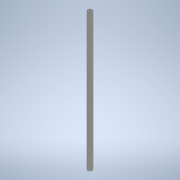
# Autodesk Inventor part: Eje
Saved by Autodesk Inventor 2020.3 (Build 243373000, 373)
## iProperties
Created: 2020-07-24
Part Number: Eje
Material: Stainless Steel
Document SubType Name: Modeling
Designer: juanp
Density: 8 g/cm^3
Appearance: Semi-Polished
Author: juanp
Autodesk Inventor part; units mm, degrees
ref_plane "YZ Plane" through (0, 0, 0) normal (1, 0, 0) x (0, 1, 0)
ref_plane "XZ Plane" through (0, 0, 0) normal (0, 1, 0) x (-1, 0, 0)
ref_plane "XY Plane" through (0, 0, 0) normal (0, 0, 1) x (1, 0, 0)
sketch "Sketch1" plane through (0, 0, 0) normal (0, 1, 0) x (-1, 0, 0)
  circle A0 centre (0, 0) radius 2.5
  dimension "d0" = 5
  constraints: 1 centre point, 1 coincident
  measures "d0" diameter of A0
extrude "Extrusion1" add sketch "Sketch1" along normal blind 152
sketch "Sketch2" plane through (0, 0, 0) normal (1, 0, 0) x (0, 1, 0)
  arc A0 (148.2919, -2.5) -> (156, -4) centre (152, -4) ccw construction
  line L0 (152, -2.5) -> (152, 2.5) projected
  line L1 (0, -2.5) -> (152, -2.5) projected
  line L2 (0, 2.5) -> (152, 2.5) projected
  arc A1 (152, 0) -> (148.2919, -2.5) centre (152, -4) ccw construction
  arc A2 (155.7081, -2.5) -> (152, 0) centre (152, -4) ccw
  line L3 (152, 0) -> (159.1444, 0) construction
  line L4 (152, -4) -> (156, -4) construction
  arc A3 (156, -4) -> (155.7081, -2.5) centre (152, -4) ccw
  point P0 (0, 0)
  dimension "d3" = 8
  constraints: 8 point on circle, 4 centre point, 4 end point, 2 horizontal, 2 midpoint, 1 point on line, 1 tangent
  measures "d3" diameter of A0
sketch "Sketch3" plane through (0, 152, 0) normal (0, 1, 0) x (1, 0, 0)
  circle A0 centre (0, 0) radius 2.5 projected
sweep "Sweep1" add profiles "Sketch3" path "Sketch2" path curves A2 A3
sketch "Sketch4" plane through (0, 156, -4) normal (0, 0, -1) x (-1, 0, 0)
  circle A0 centre (0, 0) radius 2.5 projected
  point P0 (0, -156)
extrude "Extrusion2" add sketch "Sketch4" along normal blind 10
body "Solid1"
